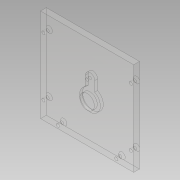
# Autodesk Inventor part: TAPA TRASERA
Saved by Autodesk Inventor 2019 (Build 230136000, 136)
## iProperties
Created: 2020-04-08
Part Number: TAPA TRASERA
Material: Plástico PMMA
Document SubType Name: Modeling
Designer: Luis Pujol
Density: 1.188 g/cm^3
Appearance: Policarbonato - Claro
Author: Luis Pujol
Autodesk Inventor part; units mm, degrees
ref_plane "YZ Plane" through (0, 0, 0) normal (1, 0, 0) x (0, 1, 0)
ref_plane "XZ Plane" through (0, 0, 0) normal (0, 1, 0) x (-1, 0, 0)
ref_plane "XY Plane" through (0, 0, 0) normal (0, 0, 1) x (1, 0, 0)
sketch "Boceto1" plane through (0, 0, 0) normal (0, 0, 1) x (1, 0, 0)
  line L0 (-80, -80) -> (80, -80)
  line L1 (80, -80) -> (80, 80)
  line L2 (80, 80) -> (-80, 80)
  line L3 (-80, 80) -> (-80, -80)
  line L4 (-80, -80) -> (80, 80) construction
  line L5 (80, -80) -> (-80, 80) construction
  circle A0 centre (0, -14.988) radius 12.5
  circle A1 centre (0, 18) radius 2.5
  point P0 (0, 0)
  dimension "d0" = 160
  dimension "d1" = 160
  dimension "d2" = 25
  dimension "d3" = 14.988
  dimension "d4" = 5
  dimension "d5" = 18
  constraints: 12 end point, 2 centre point, 2 midpoint, 2 parallel, 1 horizontal, 1 perpendicular
  measures "d0" distance of L2.end L1.end
  measures "d1" distance of L1.end L0.end
  measures "d2" diameter of A0
  measures "d3" distance of point (0, 0) A0.centre
  measures "d4" diameter of A1
  measures "d5" distance of point (0, 0) A1.centre
extrude "Extrusión1" add sketch "Boceto1" along normal blind 10
sketch "Boceto2" plane through (0, 0, 0) normal (0, 0, -1) x (-1, 0, 0)
  line L0 (80, 80) -> (80, -80) projected
  line L1 (-80, 80) -> (80, 80) projected
  line L2 (-80, -80) -> (-80, 80) projected
  line L3 (80, -80) -> (-80, -80) projected
  line L4 (-80, -80) -> (-80, 80) construction
  line L5 (-80, 0) -> (80, 0) construction
  line L6 (0, -80) -> (0, 80) construction
  line L7 (-80, 80) -> (80, 80) construction
  point P0 (0, 0)
  point P1 (75, 50)
  point P2 (75, -50)
  point P3 (50, -75)
  point P4 (-50, -75)
  point P5 (-75, 50)
  point P6 (-75, -50)
  dimension "d20" = 30
  dimension "d21" = 30
  constraints: 4 end point, 4 midpoint, 2 symmetric about line, 1 horizontal, 1 vertical, 1 other
  measures "d20" distance from line of L1 point (75, 50)
  measures "d21" distance from line of L3 point (75, -50)
hole "Agujero1" at (-75, 50, 0) at (-75, -50, 0) at (-50, -75, 0) at (50, -75, 0) at (75, -50, 0) at (75, 50, 0) direction (0, 0, 1) diameter 5.5 depth 20 tip angle 118 countersink diameter 11 countersink angle 90
sketch "Boceto3" plane through (0, 0, 0) normal (0, 0, -1) x (-1, 0, 0)
  circle A0 centre (0, -14.988) radius 12.5 projected
  circle A1 centre (0, 18) radius 2.5 projected
  arc A2 (8.0623, 18) -> (-8.0623, 18) centre (0, 18) ccw
  arc A3 (-8.0623, 0.8759) -> (8.0623, 0.8759) centre (0, -14.988) ccw
  line L0 (-8.0623, 18) -> (-8.0623, 0.8759)
  line L1 (8.0623, 18) -> (8.0623, 0.8759)
  point P0 (0, 0)
  dimension "d22" = 5.5623
  dimension "d23" = 5.2951
  constraints: 4 end point, 4 point on circle, 2 centre point, 1 vertical
  measures "d22" radial gap between concentric circles of A1 A2
  measures "d23" radial gap between concentric circles of A0 A3
extrude "Extrusión2" cut sketch "Boceto3" against normal blind 5
